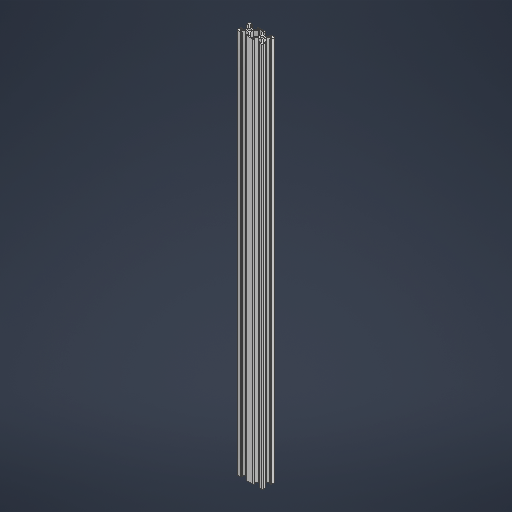
# Autodesk Inventor part: VSLOT20x40x600
Saved by Autodesk Inventor 2026.2 (Build 302298010, 298A)
## iProperties
Created: 2026-04-14
Part Number: VSLOT20x40x600
Material: Generic
Document SubType Name: Modeling
Designer: grego
Density: 1 g/cm^3
Appearance: Default
Author: grego
Autodesk Inventor part; units mm, degrees
ref_plane "YZ Plane" through (0, 0, 0) normal (1, 0, 0) x (0, 1, 0)
ref_plane "XZ Plane" through (0, 0, 0) normal (0, 1, 0) x (-1, 0, 0)
ref_plane "XY Plane" through (0, 0, 0) normal (0, 0, 1) x (1, 0, 0)
sketch "Sketch1" plane through (0, 0, 0) normal (0, 1, 0) x (-1, 0, 0)
  line L0 (3.9, -2.8393) -> (3.9, 2.8393)
  line L1 (2.8393, 3.9) -> (-2.8393, 3.9)
  line L2 (-2.8393, -3.9) -> (2.8393, -3.9)
  line L3 (8.5707, 3.2957) -> (10, 4.725)
  line L4 (8.5707, -3.2957) -> (10, -4.725)
  line L5 (8.4, 3.3664) -> (8.4, 6)
  line L6 (8.4, 6) -> (7.0607, 6)
  line L7 (10, 9) -> (10, 4.725)
  line L8 (10, -4.725) -> (10, -9)
  line L9 (3.9, 2.8393) -> (7.0607, 6)
  line L10 (3.2957, 8.5707) -> (4.725, 10)
  line L11 (3.3664, 8.4) -> (6, 8.4)
  line L12 (6, 8.4) -> (6, 7.0607)
  line L13 (2.8393, 3.9) -> (6, 7.0607)
  line L14 (8.4, -3.3664) -> (8.4, -6)
  line L15 (8.4, -6) -> (7.0607, -6)
  line L16 (3.9, -2.8393) -> (7.0607, -6)
  line L17 (3.2957, -8.5707) -> (4.725, -10)
  line L18 (3.3664, -8.4) -> (6, -8.4)
  line L19 (6, -8.4) -> (6, -7.0607)
  line L20 (2.8393, -3.9) -> (6, -7.0607)
  line L21 (-3.9, -2.8393) -> (-3.9, 2.8393)
  line L22 (-3.9, 2.8393) -> (-7.0607, 6)
  line L23 (-6, 8.4) -> (-6, 7.0607)
  line L24 (-2.8393, 3.9) -> (-6, 7.0607)
  line L25 (-3.9, -2.8393) -> (-7.0607, -6)
  line L26 (-2.8393, -3.9) -> (-6, -7.0607)
  line L27 (-6, -8.4) -> (-6, -7.0607)
  line L28 (-3.3664, -8.4) -> (-6, -8.4)
  line L29 (-3.2957, -8.5707) -> (-4.725, -10)
  line L30 (4.725, 10) -> (9, 10)
  line L31 (9, -10) -> (4.725, -10)
  circle A0 centre (0, 0) radius 2.1
  arc A1 (10, 9) -> (9, 10) centre (9, 9) ccw
  arc A2 (9, -10) -> (10, -9) centre (9, -9) ccw
  arc A3 (8.4, 3.3664) -> (8.5707, 3.2957) centre (8.5, 3.3664) ccw
  arc A4 (3.2957, 8.5707) -> (3.3664, 8.4) centre (3.3664, 8.5) ccw
  arc A5 (8.5707, -3.2957) -> (8.4, -3.3664) centre (8.5, -3.3664) ccw
  arc A6 (3.3664, -8.4) -> (3.2957, -8.5707) centre (3.3664, -8.5) ccw
  arc A7 (-3.2957, -8.5707) -> (-3.3664, -8.4) centre (-3.3664, -8.5) ccw
  line L32 (-23.9, -2.8393) -> (-23.9, 2.8393)
  line L33 (-22.8393, 3.9) -> (-17.1607, 3.9)
  line L34 (-17.1607, -3.9) -> (-22.8393, -3.9)
  line L35 (-28.5707, 3.2957) -> (-30, 4.725)
  line L36 (-28.5707, -3.2957) -> (-30, -4.725)
  line L37 (-28.4, 3.3664) -> (-28.4, 6)
  line L38 (-28.4, 6) -> (-27.0607, 6)
  line L39 (-30, 9) -> (-30, 4.725)
  line L40 (-30, -4.725) -> (-30, -9)
  line L41 (-23.9, 2.8393) -> (-27.0607, 6)
  line L42 (-23.2957, 8.5707) -> (-24.725, 10)
  line L43 (-23.3664, 8.4) -> (-26, 8.4)
  line L44 (-26, 8.4) -> (-26, 7.0607)
  line L45 (-22.8393, 3.9) -> (-26, 7.0607)
  line L46 (-23.9, 0) -> (-28.4, 0)
  line L47 (-23.9, -2.8393) -> (-27.0607, -6)
  line L48 (-28.4, -6) -> (-27.0607, -6)
  line L49 (-28.4, -3.3664) -> (-28.4, -6)
  line L50 (-22.8393, -3.9) -> (-26, -7.0607)
  line L51 (-26, -8.4) -> (-26, -7.0607)
  line L52 (-23.3664, -8.4) -> (-26, -8.4)
  line L53 (-23.2957, -8.5707) -> (-24.725, -10)
  line L54 (-16.1, -2.8393) -> (-12.9393, -6)
  line L55 (-17.1607, -3.9) -> (-14, -7.0607)
  line L56 (-16.6336, -8.4) -> (-14, -8.4)
  line L57 (-16.1, -2.8393) -> (-16.1, 2.8393)
  line L58 (-16.1, 2.8393) -> (-12.9393, 6)
  line L59 (-17.1607, 3.9) -> (-14, 7.0607)
  line L60 (-14, 8.4) -> (-14, 7.0607)
  line L61 (-14, -8.4) -> (-14, -7.0607)
  line L62 (-16.7043, -8.5707) -> (-15.275, -10)
  line L63 (-24.725, 10) -> (-29, 10)
  line L64 (-29, -10) -> (-24.725, -10)
  circle A8 centre (-20, 0) radius 2.1
  arc A9 (-29, 10) -> (-30, 9) centre (-29, 9) ccw
  arc A10 (-30, -9) -> (-29, -10) centre (-29, -9) ccw
  arc A11 (-28.5707, 3.2957) -> (-28.4, 3.3664) centre (-28.5, 3.3664) ccw
  arc A12 (-23.3664, 8.4) -> (-23.2957, 8.5707) centre (-23.3664, 8.5) ccw
  arc A13 (-28.4, -3.3664) -> (-28.5707, -3.2957) centre (-28.5, -3.3664) ccw
  arc A14 (-23.2957, -8.5707) -> (-23.3664, -8.4) centre (-23.3664, -8.5) ccw
  arc A15 (-16.6336, -8.4) -> (-16.7043, -8.5707) centre (-16.6336, -8.5) ccw
  arc A16 (-16.7043, 8.5707) -> (-16.6336, 8.4) centre (-16.6336, 8.5) ccw
  line L65 (-7.5, -8.4) -> (-7.5, -6.4393)
  line L66 (-7.0607, -6) -> (-7.5, -6.4393)
  line L67 (-12.5, -7.0607) -> (-12.5, -8.4)
  line L68 (-12.9393, -6) -> (-12.5, -6.4393)
  line L69 (-12.5, -6.4393) -> (-12.5, -7.0607)
  line L70 (-7.5, -8.4) -> (-12.5, -8.4)
  line L71 (-4.725, -10) -> (-15.275, -10)
  line L72 (-3.9, 2.8393) -> (-7.0607, 6)
  line L73 (-2.8393, 3.9) -> (-6, 7.0607)
  line L74 (-3.3664, 8.4) -> (-6, 8.4)
  line L75 (-6, 8.4) -> (-6, 7.0607)
  line L76 (-3.2957, 8.5707) -> (-4.725, 10)
  arc A17 (-3.3664, 8.4) -> (-3.2957, 8.5707) centre (-3.3664, 8.5) ccw
  line L77 (-16.1, 2.8393) -> (-12.9393, 6)
  line L78 (-17.1607, 3.9) -> (-14, 7.0607)
  line L79 (-16.6336, 8.4) -> (-14, 8.4)
  line L80 (-14, 8.4) -> (-14, 7.0607)
  line L81 (-16.7043, 8.5707) -> (-15.275, 10)
  arc A18 (-16.7043, 8.5707) -> (-16.6336, 8.4) centre (-16.6336, 8.5) ccw
  line L82 (-7.5, 8.4) -> (-7.5, 6.4393)
  line L83 (-7.0607, 6) -> (-7.5, 6.4393)
  line L84 (-12.5, 7.0607) -> (-12.5, 8.4)
  line L85 (-12.9393, 6) -> (-12.5, 6.4393)
  line L86 (-12.5, 6.4393) -> (-12.5, 7.0607)
  line L87 (-7.5, 8.4) -> (-12.5, 8.4)
  line L88 (-4.725, 10) -> (-15.275, 10)
  constraints: 178 end point, 34 point on circle, 19 centre point, 14 tangent, 5 equal radius, 4 perpendicular, 3 horizontal, 2 parallel, 1 midpoint, 1 vertical
extrude "Extrusion1" add sketch "Sketch1" along normal blind 600
body "Solid1"
